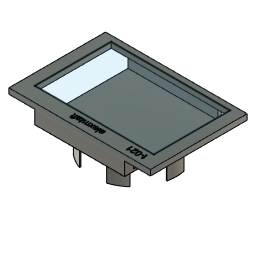
v01.01-sim-dash-g920-screen (Autodesk Fusion 360 design; units mm, degrees)
Autodesk Fusion 360 part; units mm, degrees
sketch "Sketch1" plane through (0, 0, 0) normal (0, 0, 1) x (1, 0, 0)
  line L0 (-63, 0) -> (63, 0)
  line L1 (63, 0) -> (63, -86)
  line L2 (63, -86) -> (-63, -86)
  line L3 (-63, -86) -> (-63, 0)
  dimension "d1" = 126
  dimension "d2" = 86
  constraint horizontal L0
  constraint vertical L1
  constraint horizontal L2
  constraint vertical L3
  constraint midpoint origin L0
  measures "d1" distance of L0.start L0.end
  measures "d2" distance of L0.start L2.end
extrude "Extrude1" add sketch "Sketch1" along normal blind 5
sketch "Sketch2" plane through (0, 0, 5) normal (0, 0, 1) x (-1, 0, 0)
  line L0 (63, 86) -> (-63, 86)
  line L1 (-63, 86) -> (-63, 0)
  line L2 (-63, 0) -> (63, 0)
  line L3 (63, 0) -> (63, 86)
  line L4 (53, 5) -> (-53, 5)
  line L5 (-53, 5) -> (-53, 73)
  line L6 (-53, 73) -> (53, 73)
  line L7 (53, 73) -> (53, 5)
  dimension "d5" = 106
  dimension "d6" = 68
  dimension "d8" = 10
  dimension "d9" = 5
  constraint horizontal L4
  constraint vertical L5
  constraint horizontal L6
  constraint vertical L7
  measures "d5" distance of L4.start L4.end
  measures "d6" distance of L4.end L5.end
  measures "d8" distance of L1 L5
  measures "d9" distance of L2 L4
extrude "Extrude2" cut sketch "Sketch2" against normal through all contours L4 L5 L6 L7
sketch "Sketch4" plane through (0, 0, 0) normal (0, 0, -1) x (1, 0, 0)
  line L0 (-53, 5) -> (-53, 73)
  line L1 (-53, 73) -> (53, 73)
  line L2 (53, 73) -> (53, 5)
  line L3 (53, 5) -> (-53, 5)
  line L4 (63, 86) -> (-63, 86)
  line L5 (-63, 86) -> (-63, 0)
  line L6 (-63, 0) -> (63, 0)
  line L7 (63, 0) -> (63, 86)
sketch "Sketch5" plane through (0, 0, 5) normal (0, 0, 1) x (1, 0, 0)
  line L0 (51.2778, -77.626) -> (-16.3711, -77.626) construction
  line L1 (-16.3711, -77.626) -> (-16.3711, -81.4697) construction
  line L2 (-16.3711, -81.4697) -> (51.2778, -81.4697) construction
  line L3 (51.2778, -81.4697) -> (51.2778, -77.626) construction
  dimension "d10" = 5
  text T0 "t-021           alexmtaft" font "Arial" height 5 align left top in box 67.6489 x 3.8437 at (51.2778, -77.626) x (-1, 0) y (0, -1) spacing 1 kerned
extrude "Extrude3" cut sketch "Sketch5" against normal blind 1 text T0
sketch "Sketch6" plane through (0, 0, 0) normal (0, 0, -1) x (1, 0, 0)
  line L0 (-53, 73) -> (53, 73)
  line L1 (63, 86) -> (-63, 86)
  line L2 (-40, 86) -> (40, 86)
  line L3 (40, 86) -> (40, 78)
  line L4 (40, 78) -> (-40, 78)
  line L5 (-40, 78) -> (-40, 86)
  line L6 (-40, 0) -> (40, 0)
  line L7 (40, 0) -> (40, 3)
  line L8 (40, 3) -> (-40, 3)
  line L9 (-40, 3) -> (-40, 0)
  line L10 (-63, 0) -> (63, 0)
  dimension "d13" = 8
  dimension "d14" = 80
  dimension "d15" = 3
  dimension "d16" = 80
  constraint horizontal L2
  constraint vertical L3
  constraint horizontal L4
  constraint vertical L5
  constraint midpoint L1 L2
  constraint horizontal L6
  constraint vertical L7
  constraint horizontal L8
  constraint vertical L9
  constraint midpoint L6 L10
  measures "d13" distance of L4.end L2
  measures "d14" distance of L2.start L2.end
  measures "d15" distance of L6.end L7.end
  measures "d16" distance of L7.end L8.end
extrude "Extrude4" add sketch "Sketch6" along normal blind 10
sketch "Sketch7" plane through (0, 0, -10) normal (0, 0, -1) x (1, 0, 0)
  line L0 (-40, 78) -> (40, 78)
  line L1 (40, 78) -> (40, 86)
  line L2 (40, 86) -> (-40, 86)
  line L3 (-40, 86) -> (-40, 78)
  line L4 (-40, 86) -> (40, 86)
  line L5 (40, 86) -> (40, 0)
  line L6 (40, 0) -> (-40, 0)
  line L7 (-40, 0) -> (-40, 86)
  line L8 (-63, 0) -> (63, 0)
  point P0 (40, 0)
  constraint horizontal L4
  constraint vertical L5
  constraint horizontal L6
  constraint vertical L7
  constraint coincident L2.end L3.start
  constraint coincident L6.end L8
  constraint coincident P0 L5.end
extrude "Extrude5" add sketch "Sketch7" along normal blind 2
sketch "Sketch8" plane through (0, 0, -12) normal (0, 0, -1) x (1, 0, 0)
  line L0 (-40, 0) -> (40, 0)
  line L1 (40, 0) -> (40, 86)
  line L2 (40, 86) -> (-40, 86)
  line L3 (-40, 86) -> (-40, 0)
  circle A0 centre (0, 38) radius 38
  circle A1 centre (0, 38) radius 37
  dimension "d21" = 76
  dimension "d22" = 74
  constraint concentric A0 A1
  constraint tangent L0 A0
  constraint vertical origin A0.centre
  measures "d21" diameter of A0
  measures "d22" diameter of A1
extrude "Extrude6" add sketch "Sketch8" along normal blind 25 contours A0
sketch "Sketch9" plane through (0, 0, -37) normal (0, 0, -1) x (1, 0, 0)
  circle A0 centre (0, 38) radius 37
  circle A1 centre (0, 38) radius 38
  line L0 (-12, 93.4569) -> (12, 93.4569)
  line L1 (12, 93.4569) -> (12, 63.4569)
  line L2 (12, 63.4569) -> (-12, 63.4569)
  line L3 (-12, 63.4569) -> (-12, 93.4569)
  line L4 (-28.0463, 40.3362) -> (-54.0271, 55.3362)
  line L5 (-16.0463, 61.1208) -> (-28.0463, 40.3362)
  line L6 (-42.0271, 76.1208) -> (-16.0463, 61.1208)
  line L7 (-54.0271, 55.3362) -> (-42.0271, 76.1208)
  line L8 (-16.0463, 14.8792) -> (-42.0271, -0.1208)
  line L9 (-28.0463, 35.6638) -> (-16.0463, 14.8792)
  line L10 (-54.0271, 20.6638) -> (-28.0463, 35.6638)
  line L11 (-42.0271, -0.1208) -> (-54.0271, 20.6638)
  line L12 (12, 12.5431) -> (12, -17.4569)
  line L13 (-12, 12.5431) -> (12, 12.5431)
  line L14 (-12, -17.4569) -> (-12, 12.5431)
  line L15 (12, -17.4569) -> (-12, -17.4569)
  line L16 (28.0463, 35.6638) -> (54.0271, 20.6638)
  line L17 (16.0463, 14.8792) -> (28.0463, 35.6638)
  line L18 (42.0271, -0.1208) -> (16.0463, 14.8792)
  line L19 (54.0271, 20.6638) -> (42.0271, -0.1208)
  line L20 (16.0463, 61.1208) -> (42.0271, 76.1208)
  line L21 (28.0463, 40.3362) -> (16.0463, 61.1208)
  line L22 (54.0271, 55.3362) -> (28.0463, 40.3362)
  line L23 (42.0271, 76.1208) -> (54.0271, 55.3362)
  dimension "d25" = 24
  dimension "d26" = 12
  dimension "d27" = 30
  dimension "d29" = 360
  constraint horizontal L0
  constraint vertical L1
  constraint horizontal L2
  constraint vertical L3
  measures "d25" distance of L0.start L0.end
  measures "d26" distance of A0.centre L3
  measures "d27" distance of L0.end L1.end
extrude "Extrude7" cut sketch "Sketch9" against normal up to surface (25 mm away) contours A0 A1 L20 L22 | A0 A1 L16 L18 | A0 A1 L1 L3 | A0 A1 L12 L14 | A0 A1 L4 L6 | A0 A1 L8 L10
fillet "Fillet1" radius 1 12 edges at (19, -5.091, -12) (-19, -5.091, -12) (-38, -38, -12) (-18.5, -70.0429, -12) (-19, -70.909, -12) (19, -70.909, -12) (38, -38, -12) (37, -38, -12) (18.5, -70.0429, -12) (-37, -38, -12) (-18.5, -5.9571, -12) (18.5, -5.9571, -12)
fillet "Fillet1" radius 1 12 edges at (24.7679, -66.1562, -12) (36.7679, -45.3716, -12) (24.7679, -9.8438, -12) (12, -73.5278, -12) (36.7679, -30.6284, -12) (12, -2.4722, -12) (-12, -2.4722, -12) (-36.7679, -30.6284, -12) (-36.7679, -45.3716, -12) (-12, -73.5278, -12) (-24.7679, -66.1562, -12) (-24.7679, -9.8438, -12)
